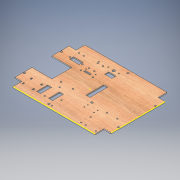
# Autodesk Inventor part: Base
Saved by Autodesk Inventor 2017 (Build 210142000, 142)
## iProperties
Created: 2017-02-09
Part Number: Base
Material: Generic
Document SubType Name: Modeling
Designer: michael
Density: 1 g/cm^3
Appearance: Default
Author: michael
Autodesk Inventor part; units mm, degrees
ref_plane "YZ Plane" through (0, 0, 0) normal (1, 0, 0) x (0, 1, 0)
ref_plane "XZ Plane" through (0, 0, 0) normal (0, 1, 0) x (-1, 0, 0)
ref_plane "XY Plane" through (0, 0, 0) normal (0, 0, 1) x (1, 0, 0)
sketch "Sketch1" plane through (0, 0, 0) normal (0, 1, 0) x (-1, 0, 0)
  line L0 (-304.8, -228.6) -> (304.8, -228.6)
  line L1 (304.8, -228.6) -> (304.8, 228.6)
  line L2 (304.8, 228.6) -> (-304.8, 228.6)
  line L3 (-304.8, 228.6) -> (-304.8, -228.6)
  line L4 (-304.8, -228.6) -> (304.8, 228.6) construction
  line L5 (304.8, -228.6) -> (-304.8, 228.6) construction
  point P0 (0, 0)
  dimension "d0" = 609.6
  dimension "d1" = 457.2
  constraints: 12 end point, 2 midpoint, 2 parallel, 1 horizontal, 1 perpendicular
  measures "d0" distance of L2.end L1.end
  measures "d1" distance of L1.end L0.end
extrude "Extrusion1" add sketch "Sketch1" along normal blind 6.35
sketch "Sketch2" plane through (0, 6.35, 0) normal (0, 1, 0) x (1, 0, 0)
  line L0 (-304.8, 228.6) -> (-304.8, -228.6) projected
  line L1 (-304.8, -228.6) -> (-260.35, -228.6)
  line L2 (-260.35, -228.6) -> (-260.35, -171.45)
  line L3 (-260.35, -171.45) -> (-304.8, -171.45)
  line L4 (-304.8, -171.45) -> (-304.8, -228.6)
  line L5 (-304.8, 228.6) -> (-260.35, 228.6)
  line L6 (-260.35, 228.6) -> (-260.35, 171.45)
  line L7 (-260.35, 171.45) -> (-304.8, 171.45)
  line L8 (-304.8, 171.45) -> (-304.8, 228.6)
  line L9 (304.8, 228.6) -> (-304.8, 228.6) projected
  line L10 (304.8, 228.6) -> (260.35, 228.6)
  line L11 (260.35, 228.6) -> (260.35, 171.45)
  line L12 (260.35, 171.45) -> (304.8, 171.45)
  line L13 (304.8, 171.45) -> (304.8, 228.6)
  line L14 (-304.8, -228.6) -> (304.8, -228.6) projected
  line L15 (304.8, -228.6) -> (260.35, -228.6)
  line L16 (260.35, -228.6) -> (260.35, -171.45)
  line L17 (260.35, -171.45) -> (304.8, -171.45)
  line L18 (304.8, -171.45) -> (304.8, -228.6)
  point P0 (0, 0)
  dimension "d4" = 44.45
  dimension "d5" = 57.15
  dimension "d6" = 44.45
  dimension "d7" = 57.15
  dimension "d8" = 44.45
  dimension "d9" = 57.15
  dimension "d10" = 44.45
  dimension "d11" = 57.15
  constraints: 32 end point, 8 parallel, 4 horizontal, 4 perpendicular
  measures "d4" distance of L3.end L2.end
  measures "d5" distance of L2.end L1.end
  measures "d6" distance of L6.end L7.end
  measures "d7" distance of L5.end L6.end
  measures "d8" distance of L12.end L11.end
  measures "d9" distance of L11.end L10.end
  measures "d10" distance of L16.end L17.end
  measures "d11" distance of L15.end L16.end
extrude "Extrusion2" cut sketch "Sketch2" against normal blind 6.35
sketch "Sketch3" plane through (0, 6.35, 0) normal (0, 1, 0) x (1, 0, 0)
  line L0 (-260.35, -228.6) -> (260.35, -228.6) projected
  line L1 (304.8, -171.45) -> (304.8, 171.45) projected
  point P0 (0, 0)
sketch "Sketch4" plane through (0, 6.35, 0) normal (0, 1, 0) x (1, 0, 0)
  line L0 (-304.8, -63.5) -> (-177.8, -63.5)
  line L1 (-177.8, -63.5) -> (-177.8, 63.5)
  line L2 (-177.8, 63.5) -> (-304.8, 63.5)
  line L3 (-304.8, 63.5) -> (-304.8, -63.5)
  line L4 (-260.35, -228.6) -> (260.35, -228.6) projected
  line L5 (260.35, 228.6) -> (-260.35, 228.6) projected
  line L6 (-304.8, 171.45) -> (-304.8, -171.45) projected
  point P0 (0, 0)
  dimension "d17" = 165.1
  dimension "d18" = 165.1
  dimension "d23" = 127
  dimension "d24" = 0
  constraints: 8 end point, 2 parallel, 1 horizontal, 1 perpendicular
  measures "d17" distance between parallel lines of L4 L0
  measures "d18" distance between parallel lines of L5 L2
  measures "d23" distance between parallel lines of L6 L1
  measures "d24" distance between parallel lines of L6 L3
extrude "Extrusion3" cut sketch "Sketch4" against normal blind 6.35
sketch "Sketch5" plane through (0, 6.35, 0) normal (0, 1, 0) x (1, 0, 0)
  circle A0 centre (-57.35, 76.2) radius 4.3
  circle A1 centre (-133.35, 76.2) radius 4.3
  circle A2 centre (-133.35, -50.8) radius 4.3
  circle A3 centre (-57.35, -50.8) radius 4.3
  line L0 (260.35, 228.6) -> (-260.35, 228.6) projected
  line L1 (-177.8, 63.5) -> (-177.8, -63.5) projected
  point P0 (0, 0)
  dimension "d25" = 8.6
  dimension "d26" = 8.6
  dimension "d27" = 8.6
  dimension "d28" = 8.6
  dimension "d29" = 127
  dimension "d30" = 127
  dimension "d31" = 152.4
  dimension "d32" = 76
  dimension "d33" = 76
  dimension "d34" = 44.45
  dimension "d35" = 44.45
  constraints: 4 centre point
  measures "d25" diameter of A0
  measures "d26" diameter of A1
  measures "d27" diameter of A2
  measures "d28" diameter of A3
  measures "d29" distance of A3.centre A0.centre
  measures "d30" distance of A2.centre A1.centre
  measures "d31" distance from line of L0 A1.centre
  measures "d32" distance of A1.centre A0.centre
  measures "d33" distance of A3.centre A2.centre
  measures "d34" distance from line of L1 A2.centre
  measures "d35" distance from line of L1 A1.centre
extrude "Extrusion4" cut sketch "Sketch5" against normal blind 25.4
sketch "Sketch6" plane through (0, 6.35, 0) normal (0, 1, 0) x (1, 0, 0)
  circle A0 centre (-204.47, 165.1) radius 4.064
  circle A1 centre (-234.95, 165.1) radius 4.064
  line L0 (-260.35, 228.6) -> (-260.35, 171.45) projected
  line L1 (260.35, 228.6) -> (-260.35, 228.6) projected
  point P0 (0, 0)
  dimension "d38" = 8.128
  dimension "d40" = 8.128
  dimension "d41" = 30.48
  dimension "d42" = 25.4
  dimension "d43" = 63.5
  dimension "d44" = 63.5
  constraints: 2 centre point
  measures "d38" diameter of A0
  measures "d40" diameter of A1
  measures "d41" distance of A0.centre A1.centre
  measures "d42" distance from line of L0 A1.centre
  measures "d43" distance from line of L1 A1.centre
  measures "d44" distance from line of L1 A0.centre
hole "Hole1" at (-204.47, 6.35, -165.1) at (-234.95, 6.35, -165.1) direction (0, -1, 0) diameter 8.128 end through all
sketch "Sketch7" plane through (0, 0, 0) normal (0, -1, 0) x (1, 0, 0)
  circle A0 centre (-161.85, -114.3) radius 4.3001
  line L0 (260.35, -228.6) -> (-260.35, -228.6) projected
  line L1 (-260.35, -171.45) -> (-260.35, -228.6) projected
  circle A1 centre (-241.3, -114.3) radius 4.3001
  line L2 (-232.081, -126.7968) -> (-171.0702, -126.7968)
  line L3 (-171.0702, -126.7968) -> (-171.0702, -101.8032)
  line L4 (-171.0702, -101.8032) -> (-232.081, -101.8032)
  line L5 (-232.081, -101.8032) -> (-232.081, -126.7968)
  line L6 (-232.081, -126.7968) -> (-171.0702, -101.8032) construction
  line L7 (-171.0702, -126.7968) -> (-232.081, -101.8032) construction
  line L8 (-177.8, -63.5) -> (-304.8, -63.5) projected
  point P0 (0, 0)
  point P1 (-201.5756, -114.3)
  dimension "d55" = 8.6002
  dimension "d90" = 8.6002
  dimension "d91" = 79.45
  dimension "d92" = 61.0108
  dimension "d93" = 24.9936
  dimension "d94" = 9.2202
  dimension "d95" = 19.05
  dimension "d96" = 50.8
  dimension "d97" = 50.8
  dimension "d98" = 50.8
  constraints: 12 end point, 2 centre point, 2 midpoint, 2 parallel, 1 horizontal, 1 perpendicular
  measures "d55" diameter of A0
  measures "d90" diameter of A1
  measures "d91" distance of A1.centre A0.centre
  measures "d92" distance of L4.end L3.end
  measures "d93" distance of L3.end L2.end
  measures "d94" distance from line of L3 A0.centre
  measures "d95" distance from line of A1.centre L1
  measures "d96" distance from line of A1.centre L8
  measures "d97" distance from line of point (-201.576, -114.3) L8
  measures "d98" distance from line of L8 A0.centre
sketch "Sketch8" plane through (0, 0, 0) normal (0, -1, 0) x (1, 0, 0)
  circle A0 centre (-86.36, -168.91) radius 4.191
  circle A1 centre (-119.38, -168.91) radius 4.191
  circle A2 centre (-86.36, -113.03) radius 4.191
  circle A3 centre (-119.38, -113.03) radius 4.191
  line L0 (260.35, -228.6) -> (-260.35, -228.6) projected
  line L1 (-177.8, 63.5) -> (-177.8, -63.5) projected
  circle A4 centre (-124.38, -180.31) radius 3.1115
  circle A5 centre (-64.38, -180.31) radius 3.1115
  circle A6 centre (-64.38, -100.31) radius 3.1115
  circle A7 centre (-124.38, -100.31) radius 3.1115
  point P0 (0, 0)
  dimension "d67" = 8.382
  dimension "d68" = 8.382
  dimension "d69" = 33.02
  dimension "d70" = 8.382
  dimension "d71" = 8.382
  dimension "d72" = 33.02
  dimension "d73" = 55.88
  dimension "d74" = 55.88
  dimension "d82" = 59.69
  dimension "d83" = 58.42
  dimension "d89" = 59.69
  dimension "d101" = 58.42
  dimension "d259" = 6.223
  dimension "d260" = 6.223
  dimension "d261" = 6.223
  dimension "d262" = 6.223
  dimension "d263" = 60
  dimension "d264" = 80
  dimension "d265" = 11.4
  dimension "d266" = 5
  dimension "d267" = 5
  dimension "d268" = 80
  dimension "d269" = 60
  constraints: 8 centre point
  measures "d67" diameter of A0
  measures "d68" diameter of A1
  measures "d69" distance of A0.centre A1.centre
  measures "d70" diameter of A2
  measures "d71" diameter of A3
  measures "d72" distance of A2.centre A3.centre
  measures "d73" distance of A1.centre A3.centre
  measures "d74" distance of A2.centre A0.centre
  measures "d82" distance from line of L0 A0.centre
  measures "d83" distance from line of L1 A3.centre
  measures "d89" distance from line of L0 A1.centre
  measures "d101" distance from line of L1 A1.centre
  measures "d259" diameter of A4
  measures "d260" diameter of A5
  measures "d261" diameter of A6
  measures "d262" diameter of A7
  measures "d263" distance of A5.centre A4.centre
  measures "d264" distance of A7.centre A4.centre
  measures "d265" vertical distance of A4.centre A1.centre
  measures "d266" horizontal distance of A4.centre A1.centre
  measures "d267" horizontal distance of A7.centre A3.centre
  measures "d268" distance of A6.centre A5.centre
  measures "d269" distance of A7.centre A6.centre
extrude "Extrusion6" cut sketch "Sketch7" against normal blind 25.4
sketch "Sketch9" plane through (0, 0, 0) normal (0, -1, 0) x (1, 0, 0)
  circle A0 centre (-27.2034, -177.8) radius 8.1153
  line L0 (260.35, -228.6) -> (-260.35, -228.6) projected
  line L1 (-260.35, -171.45) -> (-260.35, -228.6) projected
  circle A1 centre (4.5466, -177.825) radius 3.2385
  point P0 (0, 0)
  point P1 (7.7579, -178.2441)
  point P2 (7.7579, -177.4059)
  dimension "d102" = 16.2306
  dimension "d103" = 50.8
  dimension "d104" = 233.1466
  dimension "d246" = 6.477
  dimension "d250" = 31.75
  constraints: 2 centre point, 2 point on circle
  measures "d102" diameter of A0
  measures "d103" distance from line of A0.centre L0
  measures "d104" distance from line of A0.centre L1
  measures "d246" diameter of A1
  measures "d250" distance of A0.centre A1.centre
sketch "Sketch10" plane through (0, 0, 0) normal (0, -1, 0) x (1, 0, 0)
  point P0 (0, 0)
sketch "Sketch11" plane through (0, 0, 0) normal (0, -1, 0) x (1, 0, 0)
  line L0 (-36.845, -129.56) -> (8.905, -129.56)
  line L1 (8.905, -129.56) -> (8.905, -156.21)
  line L2 (8.905, -156.21) -> (-36.845, -156.21)
  line L3 (-36.845, -156.21) -> (-36.845, -129.56)
  line L4 (-36.845, -129.56) -> (8.905, -156.21) construction
  line L5 (8.905, -129.56) -> (-36.845, -156.21) construction
  line L6 (260.35, -228.6) -> (-260.35, -228.6) projected
  line L7 (-260.35, -171.45) -> (-260.35, -228.6) projected
  point P0 (0, 0)
  point P1 (-13.97, -142.885)
  dimension "d107" = 45.75
  dimension "d108" = 26.65
  dimension "d111" = 72.39
  dimension "d112" = 246.38
  constraints: 12 end point, 2 midpoint, 2 parallel, 1 horizontal, 1 perpendicular
  measures "d107" distance of L1.end L2.end
  measures "d108" distance of L0.end L1.end
  measures "d111" distance between parallel lines of L6 L2
  measures "d112" distance from line of point (-13.97, -142.885) L7
extrude "Extrusion8" cut sketch "Sketch11" against normal blind 25.4
sketch "Sketch12" plane through (0, 6.35, 0) normal (0, 1, 0) x (1, 0, 0)
  circle A0 centre (247.65, -209.55) radius 4.064
  circle A1 centre (182.65, -209.55) radius 4.064
  circle A2 centre (247.65, -74.55) radius 4.064
  circle A3 centre (182.65, -74.55) radius 4.064
  line L0 (304.8, -171.45) -> (304.8, 171.45) projected
  line L1 (-260.35, -228.6) -> (260.35, -228.6) projected
  line L2 (-260.35, -171.45) -> (-260.35, -228.6) projected
  line L3 (260.35, -228.6) -> (260.35, -171.45) projected
  point P0 (0, 0)
  dimension "d113" = 8.128
  dimension "d114" = 8.128
  dimension "d115" = 8.128
  dimension "d116" = 8.128
  dimension "d119" = 19.05
  dimension "d120" = 19.05
  dimension "d121" = 135
  dimension "d122" = 135
  dimension "d123" = 65
  dimension "d124" = 65
  dimension "d161" = 12.7
  dimension "d162" = 12.7
  constraints: 4 centre point
  measures "d113" diameter of A0
  measures "d114" diameter of A1
  measures "d115" diameter of A2
  measures "d116" diameter of A3
  measures "d119" distance from line of A0.centre L1
  measures "d120" distance from line of L1 A1.centre
  measures "d121" distance of A2.centre A0.centre
  measures "d122" distance of A1.centre A3.centre
  measures "d123" distance of A2.centre A3.centre
  measures "d124" distance of A0.centre A1.centre
  measures "d161" distance from line of L3 A0.centre
  measures "d162" distance from line of L3 A2.centre
extrude "Extrusion9" cut sketch "Sketch12" against normal blind 25.4
sketch "Sketch13" plane through (0, 6.35, 0) normal (0, 1, 0) x (1, 0, 0)
  circle A0 centre (154.4066, -209.55) radius 4.064
  line L0 (-260.35, -228.6) -> (260.35, -228.6) projected
  circle A1 centre (-31.75, -209.55) radius 4.064
  line L1 (260.35, -228.6) -> (260.35, -171.45) projected
  circle A2 centre (154.4066, -149.606) radius 4.064
  circle A3 centre (-31.75, -149.606) radius 4.064
  line L2 (-260.35, -228.6) -> (-260.35, -171.45) projected
  point P0 (0, 0)
  dimension "d127" = 8.128
  dimension "d128" = 19.05
  dimension "d129" = 8.128
  dimension "d130" = 19.05
  dimension "d131" = 186.1566
  dimension "d133" = 8.128
  dimension "d135" = 59.944
  dimension "d136" = 8.128
  dimension "d137" = 186.1566
  dimension "d138" = 59.944
  dimension "d157" = 228.6
  dimension "d158" = 228.6
  constraints: 4 centre point
  measures "d127" diameter of A0
  measures "d128" distance from line of L0 A0.centre
  measures "d129" diameter of A1
  measures "d130" distance from line of L0 A1.centre
  measures "d131" distance of A1.centre A0.centre
  measures "d133" diameter of A2
  measures "d135" distance of A2.centre A0.centre
  measures "d136" diameter of A3
  measures "d137" distance of A3.centre A2.centre
  measures "d138" distance of A1.centre A3.centre
  measures "d157" distance from line of L2 A1.centre
  measures "d158" distance from line of L2 A3.centre
extrude "Extrusion10" cut sketch "Sketch13" against normal blind 25.4
sketch "Sketch14" plane through (0, 6.35, 0) normal (0, 1, 0) x (1, 0, 0)
  point P0 (0, 0)
sketch "Sketch15" plane through (0, 6.35, 0) normal (0, 1, 0) x (1, 0, 0)
  circle A0 centre (-107.95, -180.34) radius 4.064
  circle A1 centre (-107.95, -84.6582) radius 4.064
  line L0 (260.35, -228.6) -> (260.35, -171.45) projected
  line L1 (-260.35, -228.6) -> (260.35, -228.6) projected
  line L2 (-260.35, -228.6) -> (-260.35, -171.45) projected
  point P0 (0, 0)
  dimension "d142" = 8.128
  dimension "d143" = 8.128
  dimension "d145" = 48.26
  dimension "d146" = 95.6818
  dimension "d155" = 152.4
  dimension "d156" = 152.4
  constraints: 2 centre point
  measures "d142" diameter of A0
  measures "d143" diameter of A1
  measures "d145" distance from line of L1 A0.centre
  measures "d146" distance of A1.centre A0.centre
  measures "d155" distance from line of L2 A0.centre
  measures "d156" distance from line of L2 A1.centre
extrude "Extrusion11" cut sketch "Sketch15" against normal blind 12.7
sketch "Sketch17" plane through (0, 6.35, 0) normal (0, 1, 0) x (1, 0, 0)
  line L0 (-57.15, -180.34) -> (-82.55, -180.34)
  line L1 (-82.55, -180.34) -> (-82.55, -110.0582)
  line L2 (-82.55, -110.0582) -> (-57.15, -110.0582)
  line L3 (-57.15, -110.0582) -> (-57.15, -180.34)
  circle A0 centre (-107.95, -180.34) radius 4.064 projected
  circle A1 centre (-107.95, -84.6582) radius 4.064 projected
  line L4 (-133.35, -180.34) -> (-158.75, -180.34)
  line L5 (-158.75, -180.34) -> (-158.75, -110.0582)
  line L6 (-158.75, -110.0582) -> (-133.35, -110.0582)
  line L7 (-133.35, -110.0582) -> (-133.35, -180.34)
  point P0 (0, 0)
  dimension "d163" = 0
  dimension "d164" = 25.4
  dimension "d165" = 25.4
  dimension "d166" = 25.4
  dimension "d167" = 0
  dimension "d168" = 25.4
  dimension "d169" = 25.4
  dimension "d170" = 25.4
  dimension "d171" = 25.4
  constraints: 16 end point, 4 parallel, 2 horizontal, 2 perpendicular
  measures "d163" distance from line of A0.centre L0
  measures "d164" distance from line of A1.centre L2
  measures "d165" distance from line of A1.centre L1
  measures "d166" distance of L4.start L4.end
  measures "d167" distance from line of L4 A0.centre
  measures "d168" distance from line of A1.centre L6
  measures "d169" distance from line of A1.centre L7
  measures "d170" distance between parallel lines of L5 L7
  measures "d171" distance between parallel lines of L3 L1
extrude "Extrusion13" cut sketch "Sketch17" against normal blind 12.7 contours L0 L1 L2 L3 | L4 L5 L6 L7
sketch "Sketch18" plane through (0, 0, 0) normal (0, -1, 0) x (1, 0, 0)
  line L0 (44.25, 44.45) -> (18.85, 44.45)
  line L1 (18.85, 44.45) -> (18.85, -69.85)
  line L2 (18.85, -69.85) -> (44.25, -69.85)
  line L3 (44.25, -69.85) -> (44.25, 44.45)
  circle A0 centre (-57.35, -76.2) radius 4.3 projected
  circle A1 centre (-57.35, 50.8) radius 4.3 projected
  point P0 (0, 0)
  dimension "d174" = 6.35
  dimension "d175" = 6.35
  dimension "d176" = 76.2
  dimension "d177" = 25.4
  constraints: 8 end point, 2 parallel, 1 horizontal, 1 perpendicular
  measures "d174" distance from line of A0.centre L2
  measures "d175" distance from line of L0 A1.centre
  measures "d176" distance from line of L1 A1.centre
  measures "d177" distance between parallel lines of L1 L3
extrude "Extrusion14" cut sketch "Sketch18" against normal blind 12.7 contours L3 L2 L1 L0
sketch "Sketch19" plane through (0, 6.35, 0) normal (0, 1, 0) x (1, 0, 0)
  line L0 (-241.3, -184.15) -> (-247.3607, -184.15)
  line L1 (-247.3607, -184.15) -> (-247.3607, -172.212)
  line L2 (-247.3607, -172.212) -> (-241.3, -172.212)
  line L3 (-241.3, -172.212) -> (-241.3, -184.15)
  line L4 (-176.022, -184.15) -> (-184.15, -184.15)
  line L5 (-184.15, -184.15) -> (-184.15, -172.212)
  line L6 (-184.15, -172.212) -> (-176.022, -172.212)
  line L7 (-176.022, -172.212) -> (-176.022, -184.15)
  line L8 (-260.35, -171.45) -> (-260.35, -228.6) projected
  line L9 (-260.35, -228.6) -> (260.35, -228.6) projected
  line L10 (-176.022, -132.588) -> (-184.15, -132.588)
  line L11 (-184.15, -132.588) -> (-184.15, -120.65)
  line L12 (-184.15, -120.65) -> (-176.022, -120.65)
  line L13 (-176.022, -120.65) -> (-176.022, -132.588)
  line L14 (-241.3, -132.588) -> (-249.428, -132.588)
  line L15 (-249.428, -132.588) -> (-249.428, -120.65)
  line L16 (-249.428, -120.65) -> (-241.3, -120.65)
  line L17 (-241.3, -120.65) -> (-241.3, -132.588)
  point P0 (0, 0)
  dimension "d180" = 8.128
  dimension "d181" = 76.2
  dimension "d182" = 44.45
  dimension "d183" = 11.938
  dimension "d184" = 57.15
  dimension "d185" = 11.938
  dimension "d186" = 8.128
  dimension "d187" = 8.128
  dimension "d188" = 11.938
  dimension "d189" = 76.2
  dimension "d190" = 57.15
  dimension "d191" = 63.5
  dimension "d192" = 63.5
  constraints: 32 end point, 8 parallel, 4 horizontal, 4 perpendicular, 2 point on line
  measures "d180" distance between parallel lines of L7 L5
  measures "d181" distance between parallel lines of L5 L8
  measures "d182" distance between parallel lines of L4 L9
  measures "d183" distance between parallel lines of L6 L4
  measures "d184" distance between parallel lines of L5 L3
  measures "d185" distance between parallel lines of L12 L10
  measures "d186" distance between parallel lines of L11 L13
  measures "d187" distance between parallel lines of L15 L17
  measures "d188" distance between parallel lines of L14 L16
  measures "d189" distance between parallel lines of L11 L8
  measures "d190" distance between parallel lines of L17 L11
  measures "d191" distance between parallel lines of L12 L4
  measures "d192" distance between parallel lines of L0 L16
extrude "Extrusion15" cut sketch "Sketch19" against normal blind 12.7
sketch "Sketch21" plane through (0, 6.35, 0) normal (0, 1, 0) x (1, 0, 0)
  circle A0 centre (139.7, -91.2876) radius 2.794
  circle A1 centre (78.105, -91.2876) radius 2.794
  circle A2 centre (78.105, -114.3) radius 2.794
  circle A3 centre (139.7, -114.3) radius 2.794
  line L0 (304.8, -171.45) -> (304.8, 171.45) projected
  line L1 (-260.35, -228.6) -> (260.35, -228.6) projected
  circle A4 centre (78.105, -65.8876) radius 5.8928
  point P0 (0, 0)
  dimension "d201" = 5.588
  dimension "d202" = 5.588
  dimension "d203" = 5.588
  dimension "d204" = 5.588
  dimension "d205" = 23.0124
  dimension "d206" = 61.595
  dimension "d207" = 61.595
  dimension "d208" = 165.1
  dimension "d209" = 165.1
  dimension "d210" = 23.0124
  dimension "d211" = 114.3
  dimension "d212" = 114.3
  dimension "d257" = 11.7856
  dimension "d258" = 25.4
  constraints: 5 centre point
  measures "d201" diameter of A0
  measures "d202" diameter of A1
  measures "d203" diameter of A2
  measures "d204" diameter of A3
  measures "d205" distance of A3.centre A0.centre
  measures "d206" distance of A1.centre A0.centre
  measures "d207" distance of A3.centre A2.centre
  measures "d208" distance from line of A0.centre L0
  measures "d209" distance from line of L0 A3.centre
  measures "d210" distance of A2.centre A1.centre
  measures "d211" distance from line of L1 A3.centre
  measures "d212" distance from line of L1 A2.centre
  measures "d257" diameter of A4
  measures "d258" distance of A1.centre A4.centre
sketch "Sketch22" plane through (0, 6.35, 0) normal (0, 1, 0) x (1, 0, 0)
  circle A0 centre (-298.45, 117.475) radius 5.889
  line L0 (-304.8, 171.45) -> (-304.8, 63.5) projected
  line L1 (-260.35, 171.45) -> (-304.8, 171.45) projected
  circle A1 centre (-298.45, -117.475) radius 5.889
  line L2 (-304.8, -63.5) -> (-304.8, -171.45) projected
  line L3 (-177.8, -63.5) -> (-304.8, -63.5) projected
  circle A2 centre (298.45, 117.475) radius 5.889
  line L4 (304.8, 171.45) -> (260.35, 171.45) projected
  circle A3 centre (298.45, -117.475) radius 5.889
  line L5 (260.35, -171.45) -> (304.8, -171.45) projected
  circle A4 centre (-50.8, -209.55) radius 5.889
  line L6 (-260.35, -228.6) -> (260.35, -228.6) projected
  line L7 (-260.35, -171.45) -> (-260.35, -228.6) projected
  circle A5 centre (31.75, 209.55) radius 5.889
  line L8 (-260.35, 228.6) -> (-260.35, 171.45) projected
  line L9 (260.35, 228.6) -> (-260.35, 228.6) projected
  line L10 (-304.8, 171.45) -> (-304.8, 63.5) projected
  line L11 (-304.8, -63.5) -> (-304.8, -171.45) projected
  line L12 (304.8, -171.45) -> (304.8, 171.45) projected
  point P0 (0, 0)
  dimension "d215" = 11.778
  dimension "d216" = 6.35
  dimension "d217" = 53.975
  dimension "d218" = 11.778
  dimension "d219" = 6.35
  dimension "d220" = 53.975
  dimension "d221" = 11.778
  dimension "d223" = 53.975
  dimension "d224" = 11.778
  dimension "d225" = 53.975
  dimension "d227" = 11.778
  dimension "d228" = 19.05
  dimension "d229" = 209.55
  dimension "d230" = 11.778
  dimension "d231" = 292.1
  dimension "d232" = 19.05
  dimension "d240" = 6.35
  dimension "d241" = 6.35
  constraints: 6 centre point
  measures "d215" diameter of A0
  measures "d216" distance from line of L0 A0.centre
  measures "d217" distance from line of A0.centre L1
  measures "d218" diameter of A1
  measures "d219" distance from line of L2 A1.centre
  measures "d220" distance from line of L3 A1.centre
  measures "d221" diameter of A2
  measures "d223" distance from line of L4 A2.centre
  measures "d224" diameter of A3
  measures "d225" distance from line of A3.centre L5
  measures "d227" diameter of A4
  measures "d228" distance from line of A4.centre L6
  measures "d229" distance from line of L7 A4.centre
  measures "d230" diameter of A5
  measures "d231" distance from line of L8 A5.centre
  measures "d232" distance from line of L9 A5.centre
  measures "d240" distance from line of L12 A3.centre
  measures "d241" distance from line of L12 A2.centre
extrude "Extrusion20" cut sketch "Sketch22" against normal blind 6.35
extrude "Extrusion21" cut sketch "Sketch9" against normal blind 25.4
extrude "Extrusion22" cut sketch "Sketch21" against normal blind 11.7856
extrude "Extrusion23" cut sketch "Sketch8" against normal blind 25.4
sketch "Sketch20" plane through (0, 6.35, 0) normal (0, 1, 0) x (1, 0, 0)
  line L0 (-80.01, 78.74) -> (-119.38, 78.74)
  line L1 (-119.38, 78.74) -> (-119.38, 88.9)
  line L2 (-119.38, 88.9) -> (-80.01, 88.9)
  line L3 (-80.01, 88.9) -> (-80.01, 78.74)
  circle A0 centre (-119.38, 113.03) radius 4.191 projected
  circle A1 centre (-86.36, 113.03) radius 4.191 projected
  point P0 (0, 0)
  dimension "d195" = 10.16
  dimension "d272" = 24.13
  dimension "d273" = 6.35
  constraints: 8 end point, 2 parallel, 1 horizontal, 1 perpendicular
  measures "d195" distance between parallel lines of L0 L2
  measures "d272" distance from line of A0.centre L2
  measures "d273" distance from line of L3 A1.centre
extrude "Extrusion16" cut sketch "Sketch20" against normal blind 12.7 contours L0 L1 L2 L3
equation "\"d25\" = d26"
equation "\"d27\" = d26"
equation "\"d28\" = d26"
equation "\"d30\" = d29"
equation "\"d33\" = d32"
equation "\"d35\" = d34"
equation "\"d44\" = d43"
equation "\"d90\" = d55"
equation "\"d97\" = d96"
equation "\"d98\" = d96"
equation "\"d113\" = d115"
equation "\"d114\" = d115"
equation "\"d115\" = d116"
equation "\"d120\" = d119"
equation "\"d124\" = d123"
equation "\"d162\" = d161"
equation "\"d127\" = d136"
equation "\"d129\" = d136"
equation "\"d130\" = d128"
equation "\"d133\" = d136"
equation "\"d137\" = d131"
equation "\"d138\" = d135"
equation "\"d158\" = d157"
equation "\"d142\" = d143"
equation "\"d156\" = d155"
equation "\"d164\" = d168"
equation "\"d166\" = d171"
equation "\"d168\" = d165"
equation "\"d169\" = d165"
equation "\"d185\" = d183"
equation "\"d186\" = d180"
equation "\"d187\" = d186"
equation "\"d188\" = d185"
equation "\"d189\" = d181"
equation "\"d190\" = d184"
equation "\"d201\" = d202"
equation "\"d203\" = d201"
equation "\"d204\" = d201"
equation "\"d207\" = d206"
equation "\"d209\" = d208"
equation "\"d210\" = d205"
equation "\"d212\" = d211"
equation "\"d68\" = d67"
equation "\"d70\" = d71"
equation "\"d71\" = d68"
equation "\"d72\" = d69"
equation "\"d74\" = d73"
equation "\"d101\" = d83"
body "Solid1"
